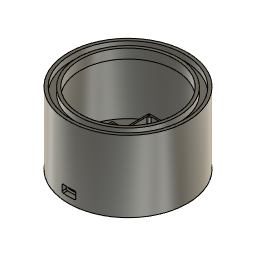
base_lamp v3 (Autodesk Fusion 360 design; units mm, degrees)
Autodesk Fusion 360 part; units mm, degrees
sketch "Boceto1" plane through (0, 0, 0) normal (0, 0, 1) x (1, 0, 0)
  circle A0 centre (0, 0) radius 50
  dimension "d4" = 100
  constraint coincident A0.centre origin
  measures "d4" diameter of A0
extrude "Extruir1" add sketch "Boceto1" along normal blind 60
sketch "Boceto2" plane through (0, 0, 60) normal (0, 0, 1) x (-1, 0, 0)
  circle A0 centre (0, 0) radius 50
  circle A1 centre (0, 0) radius 47.5
  circle A2 centre (0, 0) radius 42.5
  circle A3 centre (0, 0) radius 40
  dimension "d7" = 95
  dimension "d8" = 85
  dimension "d9" = 80
  constraint concentric A0 A1
  constraint coincident A0.centre A1.centre
  constraint concentric A2 A3
  measures "d7" diameter of A1
  measures "d8" diameter of A2
  measures "d9" diameter of A3
extrude "Extruir2" cut sketch "Boceto2" against normal blind 5 contours A1 | A3
extrude "Extruir3" cut 1 faces at (-12.741, 3.9301, 55) along direction (0, 0, -1) blind 50
sketch "Boceto3" plane through (0, 0, 5) normal (0, 0, 1) x (-1, 0, 0)
  circle A0 centre (0, 0) radius 45
  dimension "d14" = 90
  measures "d14" diameter of A0
extrude "Extruir4" cut sketch "Boceto3" along normal blind 47
sketch "Boceto4" plane through (0, 0, 5) normal (0, 0, 1) x (-1, 0, 0)
  circle A0 centre (0, 0) radius 45
  line L0 (21.5929, -21.3537) -> (-21.6071, -21.3537)
  line L1 (-21.6071, -21.3537) -> (-21.6071, -39.3537)
  line L2 (-21.6071, -39.3537) -> (21.5929, -39.3537)
  line L3 (21.5929, -39.3537) -> (21.5929, -21.3537)
  line L4 (21.5929, -21.3537) -> (-21.6071, -39.3537) construction
  line L5 (-21.6071, -21.3537) -> (21.5929, -39.3537) construction
  line L6 (20.3129, -24.5337) -> (20.3129, -36.1737)
  line L7 (-20.3271, -36.1737) -> (-20.3271, -24.5337)
  line L8 (-20.3271, -22.7337) -> (20.3129, -37.9737) construction
  line L9 (20.3129, -22.7337) -> (-20.3271, -37.9737) construction
  circle A1 centre (20.3129, -37.9737) radius 0.9
  circle A2 centre (20.3129, -22.7337) radius 0.9
  circle A3 centre (-20.3271, -22.7337) radius 0.9
  circle A4 centre (-20.3271, -37.9737) radius 0.9
  arc A5 (20.3129, -36.1737) -> (18.5129, -37.9737) centre (20.3129, -37.9737) ccw
  arc A6 (18.5129, -22.7337) -> (20.3129, -24.5337) centre (20.3129, -22.7337) ccw
  arc A7 (-20.3271, -24.5337) -> (-18.5271, -22.7337) centre (-20.3271, -22.7337) ccw
  line L10 (-18.5271, -22.7337) -> (18.5129, -22.7337)
  arc A8 (-18.5271, -37.9737) -> (-20.3271, -36.1737) centre (-20.3271, -37.9737) ccw
  line L11 (18.5129, -37.9737) -> (-18.5271, -37.9737)
  point P0 (-0.0071, -30.3537)
  point P1 (-0.0071, -30.3537)
  dimension "d17" = 43.2
  dimension "d18" = 18
  dimension "d19" = 40.64
  dimension "d20" = 15.24
  dimension "d21" = 1.8
  dimension "d22" = 1.8
  dimension "d23" = 1.8
  dimension "d24" = 1.8
  dimension "d25" = 3.6
  dimension "d28" = 3.6
  constraint horizontal L0
  constraint perpendicular L0 L1
  constraint parallel L0 L2
  constraint parallel L1 L3
  constraint coincident L4 P1
  constraint coincident L5 P1
  constraint parallel L6 L7
  constraint coincident L8 P1
  constraint coincident L9 P1
  constraint coincident P1 P0
  constraint coincident L8.end A1.centre
  constraint coincident L9.start A2.centre
  constraint coincident L8.start A3.centre
  constraint coincident L9.end A4.centre
  constraint concentric A4 A8
  measures "d17" distance of L1.end L2.end
  measures "d18" distance of L0.end L1.end
  measures "d19" distance of L8.end L9.end
  measures "d20" distance of L9.start L8.end
  measures "d21" diameter of A1
  measures "d22" diameter of A2
  measures "d23" diameter of A3
  measures "d24" diameter of A4
  measures "d25" diameter of A5
  measures "d28" diameter of A8
extrude "Extruir5" add sketch "Boceto4" along normal blind 5 contours L0 L1 L2 L3
thread "Rosca1" "ISO Metric profile 1.7 M1.7x0.35 6H" major diameter 1.7678 minor diameter 1.3711 pitch 0.35 angle 60 resizes the face on face at (-21.1033, 37.5432, 6.6667) on face at (19.5367, 37.5432, 6.6667) on face at (-21.2117, 22.7785, 8.3333) on face at (19.4283, 22.7785, 8.3333)
sketch "Boceto5" plane through (0, 0, 5) normal (0, 0, 1) x (-1, 0, 0)
  circle A0 centre (0, 0) radius 45
  line L0 (21.5929, -39.3537) -> (-21.6071, -39.3537)
  line L1 (-21.6071, -39.3537) -> (-21.6071, -21.3537)
  line L2 (-21.6071, -21.3537) -> (21.5929, -21.3537)
  line L3 (21.5929, -21.3537) -> (21.5929, -39.3537)
  line L4 (32.8916, 28.8691) -> (9.8916, 28.8691)
  line L5 (9.8916, 28.8691) -> (9.8916, -19.6309)
  line L6 (9.8916, -19.6309) -> (32.8916, -19.6309)
  line L7 (32.8916, -19.6309) -> (32.8916, 28.8691)
  line L8 (32.8916, 28.8691) -> (9.8916, -19.6309) construction
  line L9 (9.8916, 28.8691) -> (32.8916, -19.6309) construction
  line L10 (32.8916, 28.8691) -> (32.8916, 20.6691)
  line L11 (30.8916, 20.6691) -> (29.8916, 20.6691)
  line L12 (9.8916, -19.6309) -> (9.8916, -12.1309)
  circle A1 centre (29.8916, 20.6691) radius 1
  line L13 (31.3916, 27.3691) -> (11.3916, 27.3691)
  line L14 (11.3916, -18.1309) -> (31.3916, -18.1309)
  line L15 (31.3916, 27.3691) -> (11.3916, -18.1309) construction
  line L16 (11.3916, 27.3691) -> (31.3916, -18.1309) construction
  line L17 (31.3916, 18.6691) -> (29.8916, 18.6691)
  line L18 (31.3916, 22.6691) -> (29.8916, 22.6691)
  arc A2 (29.951, 22.6682) -> (29.8916, 18.6691) centre (29.8916, 20.6691) ccw
  line L19 (31.3916, -18.1309) -> (31.3916, 18.6691)
  line L20 (31.3916, 22.6691) -> (31.3916, 27.3691)
  line L21 (11.3916, 27.3691) -> (11.3916, -9.9856)
  line L22 (11.3916, -14.1309) -> (11.3916, -18.1309)
  circle A3 centre (12.8916, -12.1309) radius 1
  line L23 (11.3916, -10.1309) -> (12.8916, -10.1309)
  line L24 (11.3916, -14.1309) -> (12.8916, -14.1309)
  line L25 (11.3916, -9.9856) -> (11.3916, -10.1309)
  arc A4 (12.8916, -14.1309) -> (12.8916, -10.1309) centre (12.8916, -12.1309) ccw
  point P0 (21.3916, 4.6191)
  point P1 (21.3916, 4.6191)
  dimension "d31" = 23
  dimension "d32" = 48.5
  dimension "d33" = 8.2
  dimension "d34" = 3
  dimension "d35" = 7.5
  dimension "d38" = 2
  dimension "d39" = 20
  dimension "d40" = 45.5
  dimension "d41" = 4
  dimension "d47" = 180
  dimension "d48" = 3
  dimension "d49" = 2
  dimension "d50" = 4
  constraint horizontal L4
  constraint perpendicular L4 L5
  constraint parallel L4 L6
  constraint parallel L5 L7
  constraint coincident L8 P1
  constraint coincident L9 P1
  constraint perpendicular L4 L10
  constraint perpendicular L10 L11
  constraint perpendicular L6 L12
  constraint coincident L11.end A1.centre
  constraint horizontal L13
  constraint perpendicular L13 L21
  constraint parallel L13 L14
  constraint parallel L19 L21
  constraint coincident L15 P1
  constraint coincident L16 P1
  constraint coincident P1 P0
  constraint coincident L18.start L19
  constraint tangent L17 A2
  constraint coincident L18.end A2
  constraint coincident L8 A2.start
  constraint collinear L19 L20
  constraint coincident A1 L11.start
  constraint collinear L21 L22
  constraint parallel L22 L25
  constraint tangent L23 A4
  constraint tangent L24 A4
  measures "d31" distance of L5.end L6.end
  measures "d32" distance of L4.end L5.end
  measures "d33" distance of L4.start L10.end
  measures "d34" distance of L10.end L11.end
  measures "d35" distance of L5.end L12.end
  measures "d38" diameter of A1
  measures "d39" distance of L14.start L14.end
  measures "d40" distance of L13.end L14.start
  measures "d41" diameter of A2
  measures "d47" angle of L17 L18
  measures "d48" distance of L12.end A3.centre
  measures "d49" diameter of A3
  measures "d50" diameter of A4
extrude "Extruir6" add sketch "Boceto5" along normal blind 3.5 contours L4 L5 L6 L7 L10 L12
ref_plane "PlanoDeObra1" through (0, -50, 0) normal (0, 1, 0) x (0, 0, 1)
sketch "Boceto6" plane through (0, -50, 0) normal (0, 1, 0) x (1, 0, 0)
  line L0 (0, 0) -> (0, -5)
  line L1 (0, -5) -> (5.75, -5)
  line L2 (0, -5) -> (-5.75, -5)
  line L3 (-5.75, -5) -> (-5.75, -11.5)
  line L4 (-5.75, -11.5) -> (5.75, -11.5)
  line L5 (5.75, -11.5) -> (5.75, -5)
  line L6 (3.1, -6.95) -> (-3.1, -6.95)
  line L7 (-4.2, -8.05) -> (-4.2, -8.45)
  line L8 (-3.1, -9.55) -> (3.1, -9.55)
  line L9 (4.2, -8.45) -> (4.2, -8.05)
  line L10 (4.2, -6.95) -> (-4.2, -9.55) construction
  line L11 (-4.2, -6.95) -> (4.2, -9.55) construction
  arc A0 (-4.2, -8.45) -> (-3.1, -9.55) centre (-3.1, -8.45) ccw
  arc A1 (-3.1, -6.95) -> (-4.2, -8.05) centre (-3.1, -8.05) ccw
  arc A2 (4.2, -8.05) -> (3.1, -6.95) centre (3.1, -8.05) ccw
  arc A3 (3.1, -9.55) -> (4.2, -8.45) centre (3.1, -8.45) ccw
  point P0 (0, -8.25)
  dimension "d56" = 5
  dimension "d57" = 5.75
  dimension "d58" = 5.75
  dimension "d59" = 6.5
  dimension "d60" = 11.5
  dimension "d61" = 8.4
  dimension "d62" = 2.6
  dimension "d65" = 1.1
  dimension "d66" = 1.1
  dimension "d67" = 1.1
  dimension "d68" = 1.1
  constraint coincident L0.start origin
  constraint vertical L0
  constraint perpendicular L0 L1
  constraint perpendicular L0 L2
  constraint perpendicular L2 L3
  constraint perpendicular L3 L4
  constraint horizontal L6
  constraint perpendicular L6 L7
  constraint parallel L6 L8
  constraint parallel L7 L9
  constraint coincident L10 P0
  constraint coincident L11 P0
  constraint tangent L7 A1
  constraint tangent L6 A1
  constraint tangent L7 A0
  constraint tangent L8 A0
  constraint tangent L8 A3
  constraint tangent L9 A3
  constraint tangent L6 A2
  constraint tangent L9 A2
  measures "d56" distance of L0.start L0.end
  measures "d57" distance of L0.end L1.end
  measures "d58" distance of L0.end L2.end
  measures "d59" distance of L2.end L3.end
  measures "d60" distance of L3.end L4.end
  measures "d61" distance of L10.end L11.end
  measures "d62" distance of L11.start L10.end
  measures "d65" radius of A1
  measures "d66" radius of A0
  measures "d67" radius of A3
  measures "d68" radius of A2
extrude "Extruir7" cut sketch "Boceto6" along normal blind 3 contours L1 L2 L3 L4 L5 | L6 L7 L8 L9 A0 A1 A2 A3
sketch "Boceto7" plane through (0, -47, 0) normal (0, -1, 0) x (1, 0, 0)
  line L0 (-5.75, 5) -> (5.75, 5)
  line L1 (5.75, 5) -> (5.75, 11.5)
  line L2 (5.75, 11.5) -> (-5.75, 11.5)
  line L3 (-5.75, 11.5) -> (-5.75, 5)
  line L4 (3.1, 6.95) -> (-3.1, 6.95)
  line L5 (-4.2, 8.05) -> (-4.2, 8.45)
  line L6 (-3.1, 9.55) -> (3.1, 9.55)
  line L7 (4.2, 8.45) -> (4.2, 8.05)
  line L8 (4.2, 6.95) -> (-4.2, 9.55) construction
  line L9 (-4.2, 6.95) -> (4.2, 9.55) construction
  arc A0 (-3.1, 9.55) -> (-4.2, 8.45) centre (-3.1, 8.45) ccw
  arc A1 (-4.2, 8.05) -> (-3.1, 6.95) centre (-3.1, 8.05) ccw
  arc A2 (4.2, 8.45) -> (3.1, 9.55) centre (3.1, 8.45) ccw
  arc A3 (3.1, 6.95) -> (4.2, 8.05) centre (3.1, 8.05) ccw
  point P0 (0, 8.25)
  dimension "d71" = 8.4
  dimension "d72" = 2.6
  dimension "d73" = 1.1
  dimension "d74" = 1.1
  dimension "d75" = 1.1
  constraint horizontal L4
  constraint perpendicular L4 L5
  constraint parallel L4 L6
  constraint parallel L5 L7
  constraint coincident L8 P0
  constraint coincident L9 P0
  constraint tangent L5 A0
  constraint tangent L6 A0
  constraint tangent L5 A1
  constraint tangent L4 A1
  constraint tangent L6 A2
  constraint tangent L7 A2
  measures "d71" distance of L8.end L9.end
  measures "d72" distance of L9.start L8.end
  measures "d73" radius of A0
  measures "d74" radius of A1
  measures "d75" radius of A2
extrude "Extruir8" cut sketch "Boceto7" against normal blind 2.3 contours L4 L5 L6 L7 A0 A1 A2 A3
fillet "Empalme1" radius 1 4 edges at (-5.75, -48.3341, 11.5) (-5.75, -48.3341, 5) (5.75, -48.3341, 5) (5.75, -48.3341, 11.5)
extrude "Extruir9" cut 1 faces at (1.0333, -47, 10.85) along direction (0, 1, 0) blind 0.826
sketch "Boceto8" plane through (0, 0, 5) normal (0, 0, 1) x (-1, 0, 0)
  line L0 (21.5929, -39.3537) -> (-21.6071, -39.3537)
  line L1 (-21.6071, -39.3537) -> (-21.6071, -21.3537)
  line L2 (-21.6071, -21.3537) -> (21.5929, -21.3537)
  line L3 (21.5929, -21.3537) -> (21.5929, -39.3537)
  circle A0 centre (0, 0) radius 45
  line L4 (32.8916, -19.6309) -> (9.8916, -19.6309)
  line L5 (9.8916, -19.6309) -> (9.8916, 28.8691)
  line L6 (9.8916, 28.8691) -> (32.8916, 28.8691)
  line L7 (32.8916, 28.8691) -> (32.8916, -19.6309)
  line L8 (0, 45) -> (-5.47, 45)
  line L9 (0, 45) -> (5.47, 45)
  line L10 (-5.47, 45) -> (-5.47, 39.05)
  line L11 (-5.47, 39.05) -> (5.47, 39.05)
  line L12 (5.47, 39.05) -> (5.47, 45)
  dimension "d83" = 5.47
  dimension "d84" = 5.47
  dimension "d85" = 5.95
  dimension "d86" = 10.94
  constraint coincident A0 L8.start
  constraint perpendicular L8 L10
  constraint perpendicular L10 L11
  measures "d83" distance of L8.start L8.end
  measures "d84" distance of L8.start L9.end
  measures "d85" distance of L8.end L10.end
  measures "d86" distance of L10.end L11.end
extrude "Extruir10" add sketch "Boceto8" along normal blind 1 contours A0 L10 L11 L12 picked at (0, 41.0333)
equation "DiametroBase = 100 mm"
equation "AlturaBase = 60 mm"
equation "AlturaPantalla = 200 mm"
equation "d4 = DiametroBase"
equation "d5 = AlturaBase"
named bodies: "Base"
